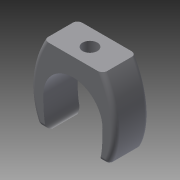
# Autodesk Inventor part: uchwyt scienny do laski
Saved by Autodesk Inventor 2014 (Build 180170000, 170)
## iProperties
Created: 2017-01-10
Part Number: uchwyt scienny do laski
Material: Ogólny
Document SubType Name: Modeling
Designer: hpdc7700
Density: 1 g/cm^3
Appearance: Domyślna
Author: hpdc7700
Autodesk Inventor part; units mm, degrees
ref_plane "YZ Plane" through (0, 0, 0) normal (1, 0, 0) x (0, 1, 0)
ref_plane "XZ Plane" through (0, 0, 0) normal (0, 1, 0) x (-1, 0, 0)
ref_plane "XY Plane" through (0, 0, 0) normal (0, 0, 1) x (1, 0, 0)
sketch "Szkic1" plane through (0, 0, 0) normal (0, 1, 0) x (-1, 0, 0)
  arc A0 (13, 0) -> (-13, 0) centre (0, 0) ccw
  line L0 (-13, 20.8683) -> (13, 20.8683)
  line L1 (-13, 20.8683) -> (-20.6231, 7.208) construction
  line L2 (-20.6231, 7.208) -> (-19.3998, -5.6367) construction
  line L3 (-19.3998, -5.6367) -> (-15.3221, -13) construction
  spline S0 degree 3 poles (-13, 20.8683) (-20.6231, 7.208) (-19.3998, -5.6367) (-15.3221, -13) knots 1 1 1 1 2 2 2 2
  line L4 (13, 20.8683) -> (20.6231, 7.208) construction
  line L5 (20.6231, 7.208) -> (19.3998, -5.6367) construction
  line L6 (19.3998, -5.6367) -> (15.3221, -13) construction
  spline S1 degree 3 poles (13, 20.8683) (20.6231, 7.208) (19.3998, -5.6367) (15.3221, -13) knots 1 1 1 1 2 2 2 2
  line L7 (-13, 0) -> (-13, -13) construction
  line L8 (-13, -13) -> (-11, -13) construction
  spline S2 degree 2 poles (-13, 0) (-13, -13) (-11, -13) knots 1 1 1 2 2 2
  line L9 (-15.3221, -13) -> (-11, -13)
  line L10 (13, 0) -> (13, -13) construction
  line L11 (13, -13) -> (11, -13) construction
  spline S3 degree 2 poles (13, 0) (13, -13) (11, -13) knots 1 1 1 2 2 2
  line L12 (15.3221, -13) -> (11, -13)
  dimension "d0" = 26
  dimension "d1" = 2
  constraints: 6 end point, 2 point on circle, 1 centre point, 1 coincident, 1 collinear, 1 horizontal, 1 parallel, 1 perpendicular, 1 tangent, 12 other
  measures "d0" diameter of A0
  measures "d1" distance of L8.end L7.end
extrude "Wyciągnięcie proste1" add sketch "Szkic1" along normal blind 15
sketch "Szkic2" plane through (-13, 0, 20.8683) normal (0, 0, 1) x (1, 0, 0)
  circle A0 centre (13, 7.5) radius 3.25
  point P0 (13, 0)
  dimension "d4" = 6.5
  constraints: 1 centre point
  measures "d4" diameter of A0
extrude "Wyciągnięcie proste2" cut sketch "Szkic2" against normal blind 15
chamfer "Faza1" distance 2 angle 45 1 edges at (-3.2497, 7.4536, 12.5873)
fillet "Zaokrąglenie1" radius 2 10 edges at (15.3221, 7.5, -13) (-15.3221, 7.5, -13) (18.5488, 15, 1.5728) (13.161, 15, -13) (-13.161, 15, -13) (-18.5488, 15, 1.5728) (13.161, 0, -13) (18.5488, 0, 1.5728) (-13.161, 0, -13) (-18.5488, 0, 1.5728)
fillet "Zaokrąglenie2" radius 2 2 edges at (-5.1418, 7.4242, 11.9399) (-3.2498, 7.4609, 14.5873)
